Wohnmobil Spacer Decker Norbert (Autodesk Fusion 360 design; units mm, degrees)
Autodesk Fusion 360 part; units mm, degrees
sketch "Sketch1" plane through (0, 0, 0) normal (0, 0, 1) x (1, 0, 0)
  line L0 (54.2564, 77.5) -> (83.7564, 77.5)
  line L1 (83.7564, 77.5) -> (83.7564, 47.5)
  line L2 (83.7564, 47.5) -> (54.2564, 47.5)
  line L3 (54.2564, 47.5) -> (54.2564, 77.5)
  line L4 (83.7564, 77.5) -> (38.7564, 77.5)
  line L5 (38.7564, 77.5) -> (38.7564, 89.5)
  line L6 (38.7564, 89.5) -> (83.7564, 89.5)
  line L7 (83.7564, 89.5) -> (83.7564, 77.5)
  dimension "d3" = 29.5
  dimension "d4" = 30
  dimension "d5" = 12
  dimension "d6" = 45
  constraint horizontal L0
  constraint vertical L1
  constraint horizontal L2
  constraint vertical L3
  constraint horizontal L4
  constraint vertical L5
  constraint horizontal L6
  constraint vertical L7
  measures "d3" distance of L1.end L2.end
  measures "d4" distance of L0.start L2.end
  measures "d5" distance of L4.end L5.end
  measures "d6" distance of L5.end L6.end
extrude "Extrude1" add sketch "Sketch1" along normal blind 4
fillet "Fillet1" radius 17 1 edges at (83.7564, 89.5, 2)
